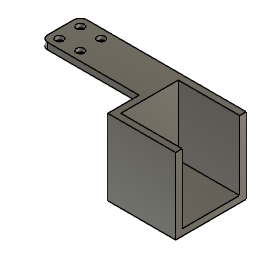
_Motor mount.2d6efdfc-5d12-4458-8d0e-ab8daa7fd196 (Autodesk Fusion 360 design; units mm, degrees)
Autodesk Fusion 360 part; units mm, degrees
sketch "Sketch1" plane through (0, 0, 0) normal (0, 0, 1) x (1, 0, 0)
  line L0 (0, 0) -> (52, 0)
  line L1 (52, 0) -> (52, -54)
  line L2 (52, -54) -> (0, -54)
  line L3 (0, -54) -> (0, 0)
  dimension "d1" = 52
  dimension "d2" = 54
  constraint horizontal L0
  constraint vertical L1
  constraint horizontal L2
  constraint vertical L3
  constraint coincident L0.start L3.end
  measures "d1" distance of L0.start L0.end
  measures "d2" distance of L0.start L2.end
extrude "Extrude1" add sketch "Sketch1" along normal blind 58
sketch "Sketch2" plane through (52, 0, 0) normal (1, 0, 0) x (0, 1, 0)
  line L0 (-54, 0) -> (0, 0)
  line L1 (0, 0) -> (0, 58)
  line L2 (0, 58) -> (-54, 58)
  line L3 (-54, 58) -> (-54, 0)
  line L4 (-5, 5) -> (-49, 5)
  line L5 (-49, 5) -> (-49, 53)
  line L6 (-49, 53) -> (-5, 53)
  line L7 (-5, 53) -> (-5, 5)
  dimension "d5" = 44
  dimension "d6" = 48
  constraint horizontal L4
  constraint vertical L5
  constraint horizontal L6
  constraint vertical L7
  measures "d5" distance of L4.start L4.end
  measures "d6" distance of L4.start L6.end
extrude "Extrude2" cut sketch "Sketch2" against normal blind 47 contours L4 L5 L6 L7
sketch "Sketch3" plane through (0, 0, 58) normal (0, 0, 1) x (-1, 0, 0)
  line L0 (0, 54) -> (-52, 54)
  line L1 (-52, 54) -> (-52, 0)
  line L2 (-52, 0) -> (0, 0)
  line L3 (0, 0) -> (0, 54)
  line L4 (-52, 5) -> (-5, 5)
  line L5 (-5, 5) -> (-5, 49)
  line L6 (-5, 49) -> (-52, 49)
  line L7 (-52, 49) -> (-52, 5)
  dimension "d9" = 47
  dimension "d10" = 44
  constraint horizontal L4
  constraint vertical L5
  constraint horizontal L6
  constraint vertical L7
  constraint coincident L1 L4.start
  measures "d9" distance of L4.start L4.end
  measures "d10" distance of L4.start L6.end
extrude "Extrude3" cut sketch "Sketch3" against normal blind 6 contours L1 L4 L5 L6 L7
sketch "Sketch4" plane through (0, 0, 58) normal (0, 0, 1) x (-1, 0, 0)
  line L0 (-5, 5) -> (-52, 5)
  line L1 (-52, 5) -> (-52, 0)
  line L2 (-52, 0) -> (0, 0)
  line L3 (0, 0) -> (0, 54)
  line L4 (0, 54) -> (-52, 54)
  line L5 (0, 0) -> (75, 0)
  line L6 (75, 0) -> (75, 30)
  line L7 (75, 30) -> (0, 30)
  line L8 (0, 30) -> (0, 0)
  line L9 (-52, 54) -> (-52, 49)
  line L10 (-52, 49) -> (-5, 49)
  line L11 (-5, 49) -> (-5, 5)
  dimension "d13" = 75
  dimension "d14" = 30
  constraint horizontal L5
  constraint vertical L6
  constraint horizontal L7
  constraint vertical L8
  constraint coincident L2.end L3.start
  measures "d13" distance of L2.end L5.end
  measures "d14" distance of L2.end L7.end
extrude "Extrude4" add sketch "Sketch4" against normal blind 5 contours L3 L5 L6 L7 L8
sketch "Sketch5" plane through (0, 0, 58) normal (0, 0, 1) x (-1, 0, 0)
  line L0 (-5, 5) -> (-52, 5)
  line L1 (-52, 5) -> (-52, 0)
  line L2 (-52, 0) -> (75, 0)
  line L3 (75, 0) -> (75, 30)
  line L4 (75, 30) -> (0, 30)
  circle A0 centre (68, 7) radius 3
  circle A1 centre (68, 23) radius 3
  circle A2 centre (52, 7) radius 3
  circle A3 centre (52, 23) radius 3
  line L5 (0, 30) -> (0, 54)
  line L6 (0, 54) -> (-52, 54)
  line L7 (-52, 54) -> (-52, 49)
  line L8 (-52, 49) -> (-5, 49)
  line L9 (-5, 49) -> (-5, 5)
  dimension "d17" = 6
  dimension "d18" = 6
  dimension "d19" = 6
  dimension "d20" = 6
  measures "d17" diameter of A0
  measures "d18" diameter of A1
  measures "d19" diameter of A2
  measures "d20" diameter of A3
extrude "Extrude5" cut sketch "Sketch5" against normal blind 5 contours A0 | A1 | A2 | A3
sketch "Sketch6" plane through (0, 0, 53) normal (0, 0, -1) x (1, 0, 0)
  circle A0 centre (-68, 23) radius 3
  circle A1 centre (-68, 7) radius 3
  circle A2 centre (-52, 23) radius 3
  circle A3 centre (-52, 7) radius 3
  line L0 (0, 0) -> (0, 30)
  line L1 (0, 30) -> (-75, 30)
  line L2 (-75, 30) -> (-75, 0)
  line L3 (-75, 0) -> (0, 0)
  circle A4 centre (-68, 23) radius 5
  circle A5 centre (-52, 23) radius 5
  circle A6 centre (-68, 7) radius 5
  circle A7 centre (-52, 7) radius 5
  dimension "d23" = 10
  dimension "d24" = 10
  dimension "d25" = 10
  dimension "d26" = 10
  constraint concentric A0 A4
  constraint concentric A2 A5
  constraint concentric A1 A6
  constraint concentric A3 A7
  measures "d23" diameter of A4
  measures "d24" diameter of A5
  measures "d25" diameter of A6
  measures "d26" diameter of A7
extrude "Extrude6" cut sketch "Sketch6" against normal blind 2 contours A4 | A5 | A6 | A7
fillet "Fillet1" radius 5 2 edges at (-75, -30, 55.5) (-75, 0, 55.5)
sketch "Sketch7" plane through (5, 0, 0) normal (1, 0, 0) x (0, 1, 0)
  line L0 (-49, 58) -> (-49, 5)
  line L1 (-49, 5) -> (-5, 5)
  line L2 (-5, 5) -> (-5, 58)
  line L3 (-5, 58) -> (-49, 58)
  line L4 (-31, 5) -> (-21, 5)
  line L5 (-21, 5) -> (-21, 15)
  line L6 (-21, 15) -> (-31, 15)
  line L7 (-31, 15) -> (-31, 5)
  dimension "d31" = 10
  dimension "d32" = 10
  constraint horizontal L4
  constraint vertical L5
  constraint horizontal L6
  constraint vertical L7
  constraint coincident L1 L4.start
  measures "d31" distance of L4.start L4.end
  measures "d32" distance of L4.start L6.end
extrude "Extrude7" cut sketch "Sketch7" against normal blind 15 contours L1 L4 L5 L6 L7
